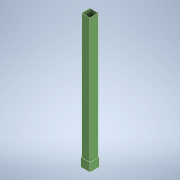
# Autodesk Inventor part: Pata_mesa
Saved by Autodesk Inventor 2021 (Build 250183000, 183)
## iProperties
Created: 2021-04-29
Part Number: Pata_mesa
Material: Genérico
Document SubType Name: Modeling
Designer: Admin
Density: 1 g/cm^3
Appearance: Default(1)
Author: Admin
Autodesk Inventor part; units mm, degrees
ref_plane "YZ Plane" through (0, 0, 0) normal (1, 0, 0) x (0, 1, 0)
ref_plane "XZ Plane" through (0, 0, 0) normal (0, 1, 0) x (-1, 0, 0)
ref_plane "XY Plane" through (0, 0, 0) normal (0, 0, 1) x (1, 0, 0)
sketch "Boceto1" plane through (0, 0, 0) normal (0, 1, 0) x (-1, 0, 0)
  line L0 (0, 0) -> (70, 0)
  line L1 (70, 0) -> (70, -70)
  line L2 (70, -70) -> (0, -70)
  line L3 (0, -70) -> (0, 0)
  line L4 (1.5, -68.5) -> (68.5, -68.5)
  line L5 (68.5, -68.5) -> (68.5, -1.5)
  line L6 (68.5, -1.5) -> (1.5, -1.5)
  line L7 (1.5, -1.5) -> (1.5, -68.5)
  line L8 (1.5, -68.5) -> (68.5, -1.5) construction
  line L9 (68.5, -68.5) -> (1.5, -1.5) construction
  point P0 (35, -35)
  dimension "d0" = 70
  dimension "d1" = 70
  dimension "d18" = 1.5
  dimension "d19" = 1.5
  dimension "d20" = 1.5
  dimension "d21" = 1.5
  constraints: 20 end point, 4 parallel, 2 horizontal, 2 midpoint, 2 perpendicular
  measures "d0" distance of L1.end L2.end
  measures "d1" distance of L0.end L1.end
  measures "d18" distance between parallel lines of L3 L7
  measures "d19" distance between parallel lines of L6 L0
  measures "d20" distance between parallel lines of L5 L1
  measures "d21" distance between parallel lines of L2 L4
extrude "Extrusión1" add sketch "Boceto1" along normal blind 1120.941
sketch "Sketch2" plane through (0, 0, 0) normal (0, -1, 0) x (1, 0, 0)
  line L0 (-70, 0) -> (0, 0) construction
  line L1 (0, 0) -> (0, -70) construction
  line L2 (0, -70) -> (-70, -70) construction
  line L3 (-70, -70) -> (-70, 0) construction
  line L4 (0, -70) -> (-70, -70) construction
  line L5 (3, 3) -> (-73, 3)
  line L6 (-73, 3) -> (-73, -73)
  line L7 (-73, -73) -> (3, -73)
  line L8 (3, -73) -> (3, 3)
  line L9 (0, -35) -> (3, -35) construction
  line L10 (-35, -70) -> (-35, -73) construction
  line L11 (-70, -35) -> (-73, -35) construction
  line L12 (-35, 0) -> (-35, 3) construction
  dimension "d10" = 3
  dimension "d11" = 3
  dimension "d12" = 3
  dimension "d13" = 3
  constraints: 16 end point, 8 midpoint, 2 horizontal, 2 parallel, 2 perpendicular, 2 vertical
  measures "d10" distance of L9.start L9.end
  measures "d11" distance of L10.start L10.end
  measures "d12" distance of L11.start L11.end
  measures "d13" distance of L12.start L12.end
extrude "Extrusion3" add sketch "Sketch2" against normal blind 70
equation "\"d0\" = d1"
equation "\"d19\" = d18"
equation "\"d20\" = d18"
equation "\"d21\" = d18"
equation "\"d11\" = d10"
equation "\"d12\" = d10"
equation "\"d13\" = d10"
